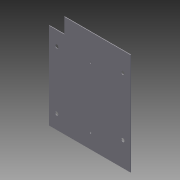
# Autodesk Inventor part: front left plate
Saved by Autodesk Inventor 2012 (Build 160160000, 160)
## iProperties
Created: 2012-03-30
Part Number: front left plate
Material: Aluminum-6061
Document SubType Name: Modeling
Designer: Edward
Density: 2.71 g/cm^3
Mass: 231.465 g
Surface Area: 1093.86 cm^2
Volume: 85.4113 cm^3
Author: Edward
Autodesk Inventor part; units mm, degrees
ref_plane "YZ Plane" through (0, 0, 0) normal (1, 0, 0) x (0, 1, 0)
ref_plane "XZ Plane" through (0, 0, 0) normal (0, 1, 0) x (-1, 0, 0)
ref_plane "XY Plane" through (0, 0, 0) normal (0, 0, 1) x (1, 0, 0)
sketch "Sketch1" plane through (0, 0, 0) normal (0, 0, 1) x (1, 0, 0)
  line L0 (0, 0) -> (213.35, 0)
  line L1 (213.35, 0) -> (213.35, 266.7)
  line L2 (213.35, 266.7) -> (0, 266.7)
  line L3 (0, 266.7) -> (0, 0)
  line L4 (0, 0) -> (41.275, 0)
  line L5 (0, 41.275) -> (0, 0)
  line L6 (0, 266.7) -> (40, 266.7)
  line L7 (40, 266.7) -> (40, 226.7)
  line L8 (40, 226.7) -> (0, 226.7)
  line L9 (0, 226.7) -> (0, 266.7)
  dimension "d0" = 266.7
  dimension "d1" = 213.35
  dimension "d4" = 40
  constraints: 20 end point, 4 parallel, 3 horizontal, 3 perpendicular
  measures "d0" distance of L2.end L0.start
  measures "d1" distance of L0.start L0.end
  measures "d4" distance of L6.end L7.end
extrude "Extrusion1" add sketch "Sketch1" along normal blind 1.5875 contours L3 L8 L7 L2 L1 L0
sketch "Sketch2" plane through (0, 0, 1.5875) normal (0, 0, 1) x (1, 0, 0)
  line L0 (213.35, 0) -> (0, 0)
  line L1 (213.35, 266.7) -> (213.35, 0)
  line L2 (40, 266.7) -> (213.35, 266.7)
  line L3 (20, 189.55) -> (20, 37.15)
  line L4 (40, 266.7) -> (40, 226.7) projected
  line L5 (40, 266.7) -> (213.35, 266.7) projected
  line L6 (0, 0) -> (0, 226.7)
  line L7 (0, 226.7) -> (40, 226.7)
  line L8 (213.35, 266.7) -> (213.35, 0) projected
  line L9 (193.35, 215.9) -> (193.35, 63.5)
  point P0 (41.275, 0)
  point P1 (126.675, 266.7)
  point P2 (20, 113.35)
  point P3 (0, 113.35)
  dimension "d9" = 152.4
  dimension "d19" = 20
  dimension "d20" = 20
  dimension "d21" = 152.4
  dimension "d22" = 50.8
  constraints: 14 end point, 3 midpoint, 2 perpendicular, 1 horizontal alignment, 1 parallel, 1 vertical alignment
  measures "d9" distance of L3.start L3.end
  measures "d19" distance between parallel lines of L6 L3
  measures "d20" distance between parallel lines of L9 L1
  measures "d21" distance of L9.start L9.end
  measures "d22" distance from line of L2 L9.start
hole "Mounting Holes" at (20, 189.55, 1.5875) at (20, 37.15, 1.5875) at (193.35, 215.9, 1.5875) at (193.35, 63.5, 1.5875) direction (0, 0, -1) diameter 8.9916 end through all clearance for "Flat Head Machine Screw" size "M8" standard "Ansi Metric M Profile"
sketch "Sketch3" plane through (0, 0, 0) normal (0, 0, -1) x (-1, 0, 0)
  line L0 (-213.35, 0) -> (-213.35, 266.7) projected
  line L1 (0, 0) -> (-213.35, 0) projected
  line L2 (0, 226.7) -> (-40, 226.7) projected
  line L3 (-108.575, 196.85) -> (-108.575, 38.1)
  dimension "d23" = 104.775
  dimension "d24" = 158.75
  dimension "d25" = 38.1
  constraints: 2 end point, 1 perpendicular
  measures "d23" distance between parallel lines of L0 L3
  measures "d24" distance of L3.start L3.end
  measures "d25" distance from line of L1 L3.end
hole "DIN Rail Holes" at (108.575, 196.85, 0) at (108.575, 38.1, 0) direction (0, 0, 1) diameter 4.4958 end through all clearance for "Flat Head Machine Screw (82)" size "#8" standard "Ansi Unified Screw Threads"
body "Solid1"
